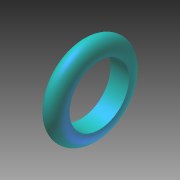
# Autodesk Inventor part: blue wheel tread
Saved by Autodesk Inventor 2012 (Build 160160000, 160)
## iProperties
Created: 2013-10-11
Part Number: blue wheel tread
Material: Default
Document SubType Name: Modeling
Designer: Bryce
Density: 1 g/cm^3
Author: Bryce
Autodesk Inventor part; units mm, degrees
ref_plane "YZ Plane" through (0, 0, 0) normal (1, 0, 0) x (0, 1, 0)
ref_plane "XZ Plane" through (0, 0, 0) normal (0, 1, 0) x (-1, 0, 0)
ref_plane "XY Plane" through (0, 0, 0) normal (0, 0, 1) x (1, 0, 0)
sketch "Sketch1" plane through (0, 0, 0) normal (0, 0, 1) x (1, 0, 0)
  line L0 (0, 0) -> (15.875, 0) construction
  line L1 (0, 25.4) -> (15.875, 25.4)
  line L2 (15.875, 25.4) -> (15.875, 26.9875)
  line L3 (15.875, 26.9875) -> (0, 26.9875) construction
  line L4 (0, 26.9875) -> (0, 25.4)
  ellipse E0 centre (7.9375, 26.9875) end of major axis (0, 26.9875) minor radius 11.1125 (15.875, 26.9875) -> (0, 26.9875) ccw
  point P0 (7.9375, 38.1)
  dimension "d0" = 1.5875
  dimension "d1" = 15.875
  dimension "d2" = 25.4
  dimension "d3" = 11.1125
  dimension "d4" = 7.9375
  dimension "d5" = 15.875
  constraints: 10 end point, 3 horizontal, 2 parallel, 1 midpoint, 1 perpendicular, 1 vertical alignment, 5 other
  measures "d0" distance of L3.end L1.start
  measures "d1" distance of L1.start L1.end
  measures "d2" distance from line of L0.start L1
  measures "d3" distance of point (7.937, 26.988) point (7.938, 38.1)
  measures "d4" distance from line of point (7.938, 38.1) L4
  measures "d5" distance of L0.start L0.end
revolve "Revolution1" add sketch "Sketch1" angle 360 about axis through (0, 0, 0) along (1, 0, 0)
equation "\"d4\" = 0.5 * d1"
equation "\"d5\" = d1"
body "Solid1"
